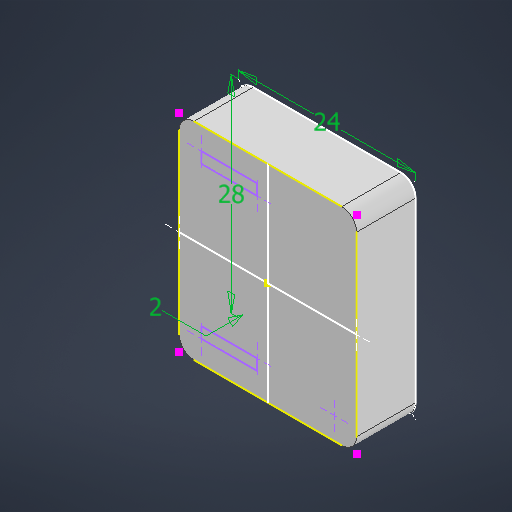
# Autodesk Inventor part: Weight_Sensor_Dummy
Saved by Autodesk Inventor 2026.2 (Build 302298010, 298A)
## iProperties
Created: 2026-03-26
Part Number: Weight_Sensor_Dummy
Material: Generic
Document SubType Name: Modeling
Designer: Srishanth Dhondy
Density: 1 g/cm^3
Appearance: Default
Author: Srishanth Dhondy
Autodesk Inventor part; units mm, degrees
ref_plane "YZ Plane" through (0, 0, 0) normal (1, 0, 0) x (0, 1, 0)
ref_plane "XZ Plane" through (0, 0, 0) normal (0, 1, 0) x (-1, 0, 0)
ref_plane "XY Plane" through (0, 0, 0) normal (0, 0, 1) x (1, 0, 0)
sketch "Sketch1" plane through (0, 0, 0) normal (0, 0, 1) x (1, 0, 0)
  line L0 (10, -14) -> (-10, -14)
  line L1 (-12, -12) -> (-12, 12)
  line L2 (-10, 14) -> (10, 14)
  line L3 (12, 12) -> (12, -12)
  line L4 (12, -14) -> (-12, 14) construction
  line L5 (-12, -14) -> (12, 14) construction
  arc A0 (-12, -12) -> (-10, -14) centre (-10, -12) ccw
  arc A1 (-10, 14) -> (-12, 12) centre (-10, 12) ccw
  arc A2 (12, 12) -> (10, 14) centre (10, 12) ccw
  arc A3 (10, -14) -> (12, -12) centre (10, -12) ccw
  point P0 (0, 0)
  dimension "d0" = 24
  dimension "d1" = 28
  dimension "d4" = 2
  constraints: 12 end point, 8 point on circle, 8 point on line, 8 tangent, 4 centre point, 3 equal radius, 2 midpoint, 2 parallel, 1 horizontal, 1 perpendicular
  measures "d0" distance of L4.end L5.end
  measures "d1" distance of L5.start L4.end
  measures "d4" radius of A0
extrude "Extrusion1" add sketch "Sketch1" along normal blind 8
sketch "Sketch2" plane through (0, 0, 8) normal (0, 0, 1) x (1, 0, 0)
  line L0 (10, 14) -> (-10, 14) projected
  line L1 (-12, 12) -> (-12, -12) projected
  line L2 (-10, -14) -> (10, -14) projected
  line L3 (12, -12) -> (12, 12) projected
  line L4 (0, 14) -> (0, -14)
  line L5 (-1.4727, -9.5234) -> (-9, -9.5234)
  line L6 (-9, -9.5234) -> (-9, -11)
  line L7 (-9, -11) -> (-1.4727, -11)
  line L8 (-1.4727, -11) -> (-1.4727, -9.5234)
  line L9 (-12, 0) -> (12, 0)
  line L10 (-12, 12) -> (-12, -12) projected
  line L11 (-1.4727, 9.5234) -> (-9, 9.5234)
  line L12 (-1.4727, 11) -> (-1.4727, 9.5234)
  line L13 (-9, 9.5234) -> (-9, 11)
  line L14 (-9, 11) -> (-1.4727, 11)
  point P0 (12, 14)
  point P1 (-12, 14)
  point P2 (-12, -14)
  point P3 (12, -14)
  point P4 (0, 0)
  point P5 (0, 0)
  point P6 (9, -11)
  constraints: 20 end point, 4 midpoint, 4 symmetric about line, 1 coincident, 1 perpendicular
body "Solid1"
